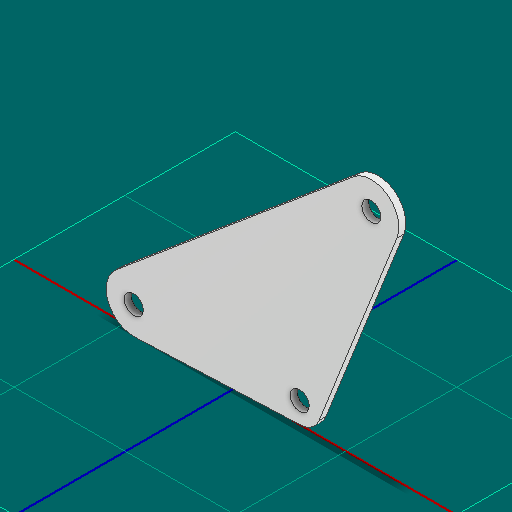
# Autodesk Inventor part: half_motor_mount
Saved by Autodesk Inventor 2025 (Build 290162000, 162)
## iProperties
Created: 2024-10-09
Part Number: half_motor_mount
Material: Acetal Resin, White
Document SubType Name: Modeling
Designer: averey
Density: 1.425 g/cm^3
Appearance: Smooth - White
Author: averey
Autodesk Inventor part; units mm, degrees
ref_plane "YZ Plane" through (0, 0, 0) normal (1, 0, 0) x (0, 1, 0)
ref_plane "XZ Plane" through (0, 0, 0) normal (0, 1, 0) x (-1, 0, 0)
ref_plane "XY Plane" through (0, 0, 0) normal (0, 0, 1) x (1, 0, 0)
sketch "main" plane through (0, 0, 0) normal (0, 0, 1) x (1, 0, 0)
  circle A0 centre (29.151, 60.8665) radius 2.1844
  circle A1 centre (29.151, 22.7665) radius 2.1844
  arc A2 (34.0093, 64.9555) -> (22.8065, 60.6019) centre (29.151, 60.8665) ccw
  arc A3 (24.3927, 22.568) -> (27.4035, 18.3362) centre (29.151, 22.7665) ccw
  circle A4 centre (74.9944, 6.3902) radius 2.1844
  arc A5 (72.6644, 0.4831) -> (79.8529, 10.4788) centre (74.9944, 6.3902) ccw
  line L0 (34.0093, 64.9555) -> (79.8529, 10.4788)
  line L1 (22.8065, 60.6019) -> (24.3927, 22.568)
  line L2 (72.6644, 0.4831) -> (27.4035, 18.3362)
  point P0 (-11.6855, 6.8462)
  point P1 (25.2705, 20.0056)
  dimension "d7" = 4.3688
  dimension "d8" = 12.7
  dimension "d9" = 9.525
  measures "d7" diameter of A4
  measures "d8" diameter of A5
  measures "d9" diameter of A3
sketch "Sketch1" plane through (0, 0, 0) normal (0, 0, 1) x (1, 0, 0)
  circle A0 centre (-21.7237, 55.4843) radius 2.1844
  circle A1 centre (16.3762, 55.4424) radius 2.1844
  arc A2 (-25.8074, 60.3471) -> (-21.4661, 49.1395) centre (-21.7237, 55.4843) ccw
  arc A3 (16.5694, 50.6838) -> (20.8046, 53.69) centre (16.3762, 55.4424) ccw
  circle A4 centre (32.803, 101.2677) radius 2.1844
  arc A5 (38.7075, 98.9311) -> (28.7197, 106.1307) centre (32.803, 101.2677) ccw
  line L0 (-25.8074, 60.3471) -> (28.7197, 106.1307)
  line L1 (-21.4661, 49.1395) -> (16.5694, 50.6838)
  line L2 (38.7075, 98.9311) -> (20.8046, 53.69)
extrude "Extrusion2" add sketch "Sketch1" along normal blind 1.5875
body "Solid2"
